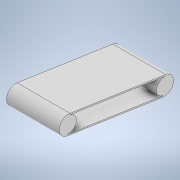
# Autodesk Inventor part: ShootingMech_Housing4
Saved by Autodesk Inventor 2020 (Build 240168000, 168)
## iProperties
Created: 2022-01-22
Part Number: ShootingMech_Housing4
Material: Generic
Document SubType Name: Modeling
Designer: danie
Density: 1 g/cm^3
Appearance: Default
Author: danie
Autodesk Inventor part; units mm, degrees
ref_plane "YZ Plane" through (0, 0, 0) normal (1, 0, 0) x (0, 1, 0)
ref_plane "XZ Plane" through (0, 0, 0) normal (0, 1, 0) x (-1, 0, 0)
ref_plane "XY Plane" through (0, 0, 0) normal (0, 0, 1) x (1, 0, 0)
sketch "Sketch1" plane through (0, 0, 0) normal (1, 0, 0) x (0, 1, 0)
  line L0 (17.213736, 115.179798) -> (-17.213736, -115.179798) construction
  line L1 (-1.627016, 117.995568) -> (-36.054488, -112.364029)
  line L2 (1.627016, -117.995568) -> (36.054488, 112.364029)
  arc A0 (36.054488, 112.364029) -> (-1.627016, 117.995568) centre (17.213736, 115.179798) ccw
  arc A1 (-36.054488, -112.364029) -> (1.627016, -117.995568) centre (-17.213736, -115.179798) ccw
  line L3 (0, 0) -> (232.918, 0) construction
  line L4 (39.194614, 111.894734) -> (4.767141, -118.464863)
  arc A2 (-39.194614, -111.894734) -> (4.767141, -118.464863) centre (-17.213736, -115.179798) ccw
  line L5 (-39.194614, -111.894734) -> (-4.767141, 118.464863)
  arc A3 (39.194614, 111.894734) -> (-4.767141, 118.464863) centre (17.213736, 115.179798) ccw
  dimension "d0" = 116.459
  dimension "d1" = 98.5
  dimension "d2" = 38.1
  dimension "d3" = 3.175
  constraints: 14 end point, 8 point on circle, 4 centre point, 4 tangent, 2 parallel, 1 equal length, 1 horizontal, 1 midpoint, 3 other
  measures "d0" distance of L3.start L0.end
  measures "d1" angle of L0 L3
  measures "d2" diameter of A1
  measures "d3" distance between parallel lines of L2 L4
extrude "Extrusion1" add sketch "Sketch1" along normal blind 127
sketch "Sketch2" plane through (127, 0, 0) normal (1, 0, 0) x (0, 0, -1)
  arc A0 (112.364029, -36.054488) -> (117.995568, 1.627016) centre (115.179798, -17.213736) ccw
  ellipse E0 centre (115.179798, -17.213736) end of major axis (117.995568, 1.627016) minor radius 19.05
  arc A1 (-111.894734, 39.194614) -> (-118.464863, -4.767141) centre (-115.179798, 17.213736) ccw
  arc A2 (-112.364029, 36.054488) -> (-117.995568, -1.627016) centre (-115.179798, 17.213736) ccw
  ellipse E1 centre (-115.179798, 17.213736) end of major axis (-112.364029, 36.054488) minor radius 19.05
  point P0 (0, 0)
  constraints: 2 coincident, 6 other
extrude "Extrusion2" add sketch "Sketch2" against normal blind 127
body "Solid1"
